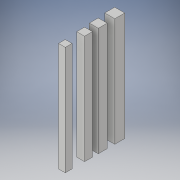
# Autodesk Inventor part: Part2
Saved by Autodesk Inventor 2018 (Build 220112000, 112)
## iProperties
Created: 2018-01-23
Part Number: Part2
Material: Generic
Document SubType Name: Modeling
Designer: prakh
Density: 1 g/cm^3
Appearance: Default
Author: prakh
Autodesk Inventor part; units mm, degrees
ref_plane "YZ Plane" through (0, 0, 0) normal (1, 0, 0) x (0, 1, 0)
ref_plane "XZ Plane" through (0, 0, 0) normal (0, 1, 0) x (-1, 0, 0)
ref_plane "XY Plane" through (0, 0, 0) normal (0, 0, 1) x (1, 0, 0)
sketch "Sketch1" plane through (0, 0, 0) normal (0, 1, 0) x (-1, 0, 0)
  line L0 (0.6048, -3.1754) -> (3.7798, -3.1754)
  line L1 (3.7798, -3.1754) -> (3.7798, -6.3504)
  line L2 (3.7798, -6.3504) -> (0.6048, -6.3504)
  line L3 (0.6048, -6.3504) -> (0.6048, -3.1754)
  line L4 (0.6048, -12.2) -> (4.2878, -12.2)
  line L5 (4.2878, -12.2) -> (4.2878, -15.883)
  line L6 (4.2878, -15.883) -> (0.6048, -15.883)
  line L7 (0.6048, -15.883) -> (0.6048, -12.2)
  line L8 (0.6048, -18.5938) -> (4.7958, -18.5938)
  line L9 (4.7958, -18.5938) -> (4.7958, -22.7848)
  line L10 (4.7958, -22.7848) -> (0.6048, -22.7848)
  line L11 (0.6048, -22.7848) -> (0.6048, -18.5938)
  line L12 (0.6048, -26.303) -> (5.3038, -26.303)
  line L13 (5.3038, -26.303) -> (5.3038, -31.002)
  line L14 (5.3038, -31.002) -> (0.6048, -31.002)
  line L15 (0.6048, -31.002) -> (0.6048, -26.303)
  point P0 (0, 0)
  point P1 (2.1923, -4.7629)
  point P2 (2.4463, -14.0415)
  point P3 (2.7003, -20.6893)
  point P4 (2.9543, -28.6525)
  dimension "d0" = 3.175
  dimension "d1" = 3.683
  dimension "d2" = 4.191
  dimension "d3" = 4.699
  constraints: 32 end point, 4 horizontal, 3 vertical alignment, 36 other
  measures "d0" distance of L0.end L1.end
  measures "d1" distance of L4.end L5.end
  measures "d2" distance of L8.end L9.end
  measures "d3" distance of L12.end L13.end
extrude "Extrusion1" add sketch "Sketch1" along normal blind 50.8
body "Solid1"
